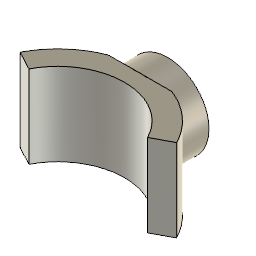
penplotter_attchment v4 (Autodesk Fusion 360 design; units mm, degrees)
Autodesk Fusion 360 part; units mm, degrees
sketch "スケッチ1" plane through (0, 0, 0) normal (0, 0, 1) x (1, 0, 0)
  line L0 (-5.3799, 2.7675) -> (-7.1041, 3.6785)
  line L1 (5.3799, 2.7675) -> (7.1041, 3.6785)
  line L2 (-2.8572, 7.4724) -> (2.8572, 7.4724)
  arc A0 (5.3799, 2.7675) -> (-5.3799, 2.7675) centre (0, 0) ccw
  arc A1 (7.1041, 3.6785) -> (2.8572, 7.4724) centre (0, 0) ccw
  arc A2 (-2.8572, 7.4724) -> (-7.1041, 3.6785) centre (0, 0) ccw
  dimension "d1" = 12.1
  constraint coincident A0.centre A1.centre
  constraint concentric A0 A1
  constraint coincident L2.start A1
  constraint horizontal L2
  constraint concentric A1 A2
  measures "d1" diameter of A0
extrude "押し出し1" add sketch "スケッチ1" along normal blind 7.5
sketch "スケッチ4" plane through (0, 7.4724, 0) normal (0, 1, 0) x (-1, 0, 0)
  line L0 (-2.8572, 0) -> (2.8572, 0)
  line L1 (2.8572, 0) -> (2.8572, 7.5)
  line L2 (2.8572, 7.5) -> (-2.8572, 7.5)
  line L3 (-2.8572, 7.5) -> (-2.8572, 0)
  line L4 (0, 7.5) -> (0, 0)
  line L5 (0, 0.5746) -> (2.75, 2.1623)
  line L6 (2.75, 2.1623) -> (2.75, 5.3377)
  line L7 (2.75, 5.3377) -> (0, 6.9254)
  line L8 (0, 6.9254) -> (-2.75, 5.3377)
  line L9 (-2.75, 5.3377) -> (-2.75, 2.1623)
  line L10 (-2.75, 2.1623) -> (0, 0.5746)
  circle A0 centre (0, 3.75) radius 3.75
  point P0 (0, 3.75)
  dimension "d12" = 5.5
  constraint midpoint L2 L4.start
  constraint coincident L4.end origin
  constraint coincident L4 L5.start
  constraint midpoint L4 P0
  constraint coincident P0 A0.centre
  measures "d12" distance of L7 L10
extrude "押し出し4" add sketch "スケッチ4" along normal blind 2.5 contours L3 L4 L8 L9 L10 A0 | L1 L4 L5 L6 L7 A0 | L3 A0 | L1 A0
